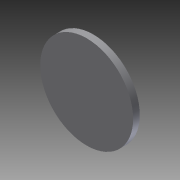
# Autodesk Inventor part: panProjectorGear
Saved by Autodesk Inventor 2012 (Build 160160000, 160)
## iProperties
Created: 2014-06-12
Part Number: panProjectorGear
Material: Default
Document SubType Name: Modeling
Designer: Byron
Density: 1 g/cm^3
Author: Byron
Autodesk Inventor part; units mm, degrees
ref_plane "YZ Plane" through (0, 0, 0) normal (1, 0, 0) x (0, 1, 0)
ref_plane "XZ Plane" through (0, 0, 0) normal (0, 1, 0) x (-1, 0, 0)
ref_plane "XY Plane" through (0, 0, 0) normal (0, 0, 1) x (1, 0, 0)
sketch "Sketch1" plane through (0, 0, 0) normal (0, 0, 1) x (1, 0, 0)
  line L0 (-34.7671, 44.45) -> (-55.7204, 44.45) projected
  line L1 (-45.2437, 44.45) -> (-45.2437, -51.1902) construction
  circle A0 centre (10.6363, 0) radius 3.175 construction
  line L2 (10.6363, 0) -> (-76.563, 0) construction
  circle A1 centre (-45.2437, 32.6782) radius 44.45
  point P0 (0, 0)
  dimension "d0" = 88.9
  constraints: 4 end point, 2 perpendicular, 1 centre point, 1 midpoint, 1 point on line
  measures "d0" diameter of A1
extrude "Extrusion1" add sketch "Sketch1" along normal blind 6.35
body "Solid1"
